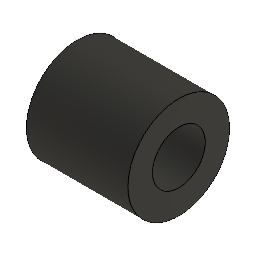
ServoBox (Autodesk Fusion 360 archive; units mm, degrees)
design "0.375 OD Spacer, 0.375 (Nylon)"
Autodesk Fusion 360 part; units mm, degrees
note: some values were not read from the file. Chosen so that the rebuilt part matches the saved one: a direction; which face or edge a step refers to. Set by a fixed rule: which sketch regions a step uses.
(part 1 of 2)
sketch "sketch 165" plane through (0, 0, 0) normal (1, 0, 0) x (0, 1, 0)
  circle A0 centre (0, 0) radius 4.7625
  circle A1 centre (0, 0) radius 2.4638
extrude "Extrude1" add sketch "sketch 165" along normal blind 9.525

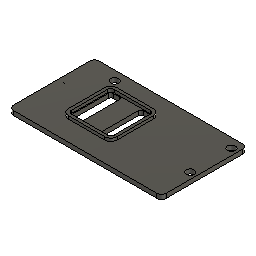
design "Encoder Mount"
Autodesk Fusion 360 part; units mm, degrees
sketch "Sketch1" plane through (0, 0, 0) normal (0, 0, 1) x (1, 0, 0)
  circle A0 centre (18.7728, 42.4051) radius 2.159
  line L0 (-60.9197, 30.0451) -> (-60.9197, 58.9153)
  line L1 (22.2603, 30.0451) -> (22.2603, 58.9153)
  circle A1 centre (-44.7272, 19.9053) radius 2.159
  circle A2 centre (18.7728, 19.9051) radius 2.159
  line L2 (-60.9197, 30.0451) -> (-60.9197, 17.3451)
  line L3 (22.2603, 30.0451) -> (22.2603, 17.3451)
  line L4 (19.7203, 14.8051) -> (3.2103, 14.8051)
  line L5 (-41.8697, 14.8051) -> (-58.3797, 14.8051)
  arc A3 (-60.9197, 17.3451) -> (-58.3797, 14.8051) centre (-58.3797, 17.3451) ccw
  arc A4 (19.7203, 14.8051) -> (22.2603, 17.3451) centre (19.7203, 17.3451) ccw
  line L6 (-41.8697, 14.8051) -> (3.2103, 14.8051)
  line L7 (-57.4272, 61.4553) -> (19.7203, 61.4553)
  line L8 (-57.4272, 61.4553) -> (-58.3797, 61.4553)
  arc A5 (-58.3797, 61.4553) -> (-60.9197, 58.9153) centre (-58.3797, 58.9153) ccw
  arc A6 (22.2603, 58.9153) -> (19.7203, 61.4553) centre (19.7203, 58.9153) ccw
  line L9 (-23.0468, 48.4378) -> (-19.6337, 48.4378)
  line L10 (-18.3637, 47.1678) -> (-18.3637, 27.4828)
  line L11 (-40.5887, 27.4828) -> (-40.5887, 47.1678)
  line L12 (-39.3187, 48.4378) -> (-35.9056, 48.4378)
  line L13 (-57.7726, 34.7366) -> (-57.0819, 34.7366)
  line L14 (-34.6356, 38.3051) -> (-34.6356, 47.1678)
  line L15 (-34.6356, 38.3051) -> (-34.6356, 27.4828)
  line L16 (-24.3168, 38.3051) -> (-24.3168, 47.1678)
  line L17 (-24.3168, 38.3051) -> (-24.3168, 27.4828)
  line L18 (-19.6337, 26.2128) -> (-23.0468, 26.2128)
  line L19 (-35.9056, 26.2128) -> (-39.3187, 26.2128)
  arc A7 (-39.3187, 48.4378) -> (-40.5887, 47.1678) centre (-39.3187, 47.1678) ccw
  arc A8 (-34.6356, 47.1678) -> (-35.9056, 48.4378) centre (-35.9056, 47.1678) ccw
  arc A9 (-23.0468, 48.4378) -> (-24.3168, 47.1678) centre (-23.0468, 47.1678) ccw
  arc A10 (-18.3637, 47.1678) -> (-19.6337, 48.4378) centre (-19.6337, 47.1678) ccw
  arc A11 (-19.6337, 26.2128) -> (-18.3637, 27.4828) centre (-19.6337, 27.4828) ccw
  arc A12 (-24.3168, 27.4828) -> (-23.0468, 26.2128) centre (-23.0468, 27.4828) ccw
  arc A13 (-35.9056, 26.2128) -> (-34.6356, 27.4828) centre (-35.9056, 27.4828) ccw
  arc A14 (-40.5887, 27.4828) -> (-39.3187, 26.2128) centre (-39.3187, 27.4828) ccw
  line L20 (-40.5887, 37.3253) -> (-60.9087, 37.3253)
  line L21 (-37.6121, 48.4378) -> (-37.6121, 61.4553)
  arc A15 (-57.0819, 34.7366) -> (-57.7726, 34.7366) centre (-57.4272, 32.6053) ccw
  point P0 (-54.3297, 57.5051)
  point P1 (-60.9197, 27.5051)
  point P2 (-60.9197, 71.9551)
  point P3 (22.2603, 27.5051)
  point P4 (22.2603, 71.9551)
  point P5 (-60.9197, 14.8051)
  point P6 (22.2603, 14.8051)
  point P7 (-18.3637, 48.4378)
  point P8 (-18.3637, 26.2128)
  point P9 (-40.5887, 26.2128)
  point P10 (-40.5887, 48.4378)
  dimension "d37" = 4.318
  dimension "d42" = 4.318
  dimension "d49" = 44.45
  dimension "d51" = 44.45
  dimension "d84" = 4.318
  dimension "d86" = 4.318
  dimension "d89" = 15.24
  dimension "d90" = 15.24
  dimension "d93" = 2.54
  dimension "d139" = 2.54
  dimension "d142" = 22.225
  dimension "d143" = 22.225
  dimension "d144" = 22.225
  dimension "d146" = 10.3188
  dimension "d149" = 1.27
  dimension "d155" = 20.32
  dimension "d156" = 13.0175
  constraint coincident P2 L0
  constraint coincident P4 L1
  constraint coincident P3 L1
  constraint coincident P1 L0
  constraint collinear L4 L5
  constraint coincident P5 L2
  constraint coincident P5 L5
  constraint tangent L2 A3
  constraint tangent L5 A3
  constraint coincident P6 L3
  constraint coincident P6 L4
  constraint tangent L3 A4
  constraint tangent L4 A4
  constraint equal A3 A4
  constraint perpendicular L0 L13
  constraint perpendicular L1 L7
  constraint perpendicular L0 L8
  constraint tangent L8 A5
  constraint tangent L0 A5
  constraint tangent L7 A6
  constraint tangent L1 A6
  constraint equal A5 A6
  constraint perpendicular L9 L10
  constraint perpendicular L10 L18
  constraint perpendicular L11 L18
  constraint perpendicular L7 L14
  constraint perpendicular L6 L15
  constraint perpendicular L7 L16
  constraint perpendicular L6 L17
  constraint collinear L18 L19
  constraint coincident P10 L11
  constraint coincident P10 L12
  constraint tangent L11 A7
  constraint tangent L12 A7
  constraint tangent L14 A8
  constraint tangent L12 A8
  constraint equal A7 A8
  constraint tangent L16 A9
  constraint tangent L9 A9
  constraint equal A7 A9
  constraint coincident P7 L9
  constraint coincident P7 L10
  constraint tangent L9 A10
  constraint tangent L10 A10
  constraint equal A7 A10
  constraint coincident P8 L10
  constraint coincident P8 L18
  constraint tangent L10 A11
  constraint tangent L18 A11
  constraint equal A7 A11
  constraint tangent L18 A12
  constraint tangent L17 A12
  constraint equal A7 A12
  constraint tangent L19 A13
  constraint tangent L15 A13
  constraint equal A7 A13
  constraint coincident P9 L19
  constraint coincident P9 L11
  constraint tangent L19 A14
  constraint tangent L11 A14
  constraint equal A7 A14
  constraint midpoint L11 L20.start
  constraint perpendicular L0 L20
  constraint midpoint L12 L21.start
  constraint perpendicular L7 L21
  constraint coincident L7 L21.end
  measures "d37" diameter of A0
  measures "d42" diameter of A15
  measures "d49" distance of P1 P2
  measures "d51" distance of P3 P4
  measures "d84" diameter of A1
  measures "d86" diameter of A2
  measures "d89" distance of L0.start P5
  measures "d90" distance of L1.start P6
  measures "d93" radius of A3
  measures "d139" radius of A5
  measures "d142" distance of P7 P8
  measures "d143" distance of P8 P9
  measures "d144" distance of P9 P10
  measures "d146" distance of L16.start L14.start
  measures "d149" radius of A7
  measures "d155" distance of L20.start L20.end
  measures "d156" distance of L21.start L21.end
extrude "Extrude11" add sketch "Sketch1" along normal blind 2.3813
sketch "Sketch10" plane through (0, 0, 2.3813) normal (0, 0, 1) x (-1, 0, 0)
  circle A0 centre (44.7272, -19.9053) radius 2.159
  circle A1 centre (-18.7728, -19.9051) radius 2.159
  circle A2 centre (-18.7728, -42.4051) radius 2.159
  line L0 (24.3168, -27.4828) -> (24.3168, -47.1678)
  line L1 (23.0468, -48.4378) -> (19.6337, -48.4378)
  line L2 (18.3637, -47.1678) -> (18.3637, -27.4828)
  line L3 (35.9056, -26.2128) -> (39.3187, -26.2128)
  line L4 (34.6356, -47.1678) -> (34.6356, -27.4828)
  line L5 (40.5887, -27.4828) -> (40.5887, -47.1678)
  line L6 (39.3187, -48.4378) -> (35.9056, -48.4378)
  line L7 (-22.2603, -17.3451) -> (-22.2603, -58.9153)
  arc A3 (-22.2603, -58.9153) -> (-19.7203, -61.4553) centre (-19.7203, -58.9153) ccw
  line L8 (-19.7203, -61.4553) -> (58.3797, -61.4553)
  arc A4 (58.3797, -61.4553) -> (60.9197, -58.9153) centre (58.3797, -58.9153) ccw
  line L9 (60.9197, -58.9153) -> (60.9197, -17.3451)
  arc A5 (60.9197, -17.3451) -> (58.3797, -14.8051) centre (58.3797, -17.3451) ccw
  line L10 (58.3797, -14.8051) -> (-19.7203, -14.8051)
  arc A6 (-19.7203, -14.8051) -> (-22.2603, -17.3451) centre (-19.7203, -17.3451) ccw
  arc A7 (39.3187, -48.4378) -> (40.5887, -47.1678) centre (39.3187, -47.1678) ccw
  arc A8 (34.6356, -47.1678) -> (35.9056, -48.4378) centre (35.9056, -47.1678) ccw
  arc A9 (35.9056, -26.2128) -> (34.6356, -27.4828) centre (35.9056, -27.4828) ccw
  arc A10 (40.5887, -27.4828) -> (39.3187, -26.2128) centre (39.3187, -27.4828) ccw
  arc A11 (23.0468, -48.4378) -> (24.3168, -47.1678) centre (23.0468, -47.1678) ccw
  arc A12 (18.3637, -47.1678) -> (19.6337, -48.4378) centre (19.6337, -47.1678) ccw
  arc A13 (19.6337, -26.2128) -> (18.3637, -27.4828) centre (19.6337, -27.4828) ccw
  line L11 (19.6337, -26.2128) -> (23.0468, -26.2128)
  arc A14 (24.3168, -27.4828) -> (23.0468, -26.2128) centre (23.0468, -27.4828) ccw
  line L12 (39.3264, -48.4391) -> (19.6414, -48.4391)
  line L13 (18.3714, -47.1691) -> (18.3714, -27.4841)
  line L14 (19.6414, -26.2141) -> (39.3264, -26.2141)
  line L15 (40.5964, -27.4841) -> (40.5964, -47.1691)
  arc A15 (39.3264, -48.4391) -> (40.5964, -47.1691) centre (39.3264, -47.1691) ccw
  arc A16 (18.3714, -47.1691) -> (19.6414, -48.4391) centre (19.6414, -47.1691) ccw
  arc A17 (19.6414, -26.2141) -> (18.3714, -27.4841) centre (19.6414, -27.4841) ccw
  arc A18 (40.5964, -27.4841) -> (39.3264, -26.2141) centre (39.3264, -27.4841) ccw
  line L16 (19.6414, -25.6849) -> (39.3264, -25.6849)
  arc A19 (41.1255, -27.4841) -> (39.3264, -25.6849) centre (39.3264, -27.4841) ccw
  line L17 (41.1255, -27.4841) -> (41.1255, -47.1691)
  arc A20 (39.3264, -48.9683) -> (41.1255, -47.1691) centre (39.3264, -47.1691) ccw
  line L18 (39.3264, -48.9683) -> (19.6414, -48.9683)
  arc A21 (17.8422, -47.1691) -> (19.6414, -48.9683) centre (19.6414, -47.1691) ccw
  line L19 (17.8422, -47.1691) -> (17.8422, -27.4841)
  arc A22 (19.6414, -25.6849) -> (17.8422, -27.4841) centre (19.6414, -27.4841) ccw
  arc A23 (16.2547, -47.1691) -> (19.6414, -50.5558) centre (19.6414, -47.1691) ccw
  line L20 (39.3264, -50.5558) -> (19.6414, -50.5558)
  arc A24 (39.3264, -50.5558) -> (42.713, -47.1691) centre (39.3264, -47.1691) ccw
  line L21 (42.713, -27.4841) -> (42.713, -47.1691)
  arc A25 (42.713, -27.4841) -> (39.3264, -24.0974) centre (39.3264, -27.4841) ccw
  line L22 (19.6414, -24.0974) -> (39.3264, -24.0974)
  arc A26 (19.6414, -24.0974) -> (16.2547, -27.4841) centre (19.6414, -27.4841) ccw
  line L23 (16.2547, -47.1691) -> (16.2547, -27.4841)
  arc A27 (57.0819, -34.7366) -> (57.7726, -34.7366) centre (57.4272, -32.6053) ccw
  line L24 (57.0819, -34.7366) -> (57.7726, -34.7366)
  dimension "d150" = -0.5292
  dimension "d151" = 1.27
  dimension "d154" = -1.5875
  constraint perpendicular L2 L12
  constraint perpendicular L11 L13
  constraint perpendicular L5 L14
  constraint perpendicular L12 L15
  constraint tangent L12 A15
  constraint tangent L15 A15
  constraint tangent L12 A16
  constraint tangent L13 A16
  constraint equal A15 A16
  constraint tangent L13 A17
  constraint tangent L14 A17
  constraint equal A15 A17
  constraint tangent L14 A18
  constraint tangent L15 A18
  constraint equal A15 A18
  measures "d151" radius of A15
extrude "Extrude12" add sketch "Sketch10" against normal blind 3.9688 contours A23 L20 A24 L21 A25 L22 A26 L23
move_body "Move1" bodies 1 to x (1, 0, 0) y (0, -1, 0) z (0, 0, -1) at (0, 51.5532, 4.7625)
equation "d142 = ( 7 / 8 ) * 1 in"
equation "d143 = ( 7 / 8 ) * 1 in"
equation "d144 = ( 7 / 8 ) * 1 in"
equation "d146 = ( 13 / 32 ) * 1 in"
equation "d147 = ( 3 / 32 ) * 1 in"
equation "d150 = ( -1 / 48 ) * 1 in"
equation "d152 = ( -5 / 32 ) * 1 in"
equation "d154 = ( -1 / 16 ) * 1 in"
equation "d120 = ( 3 / 16 ) * 1 in"
equation "d122 = 2.04724 in + 0.375 in"
equation "d123 = ( 3 / 16 ) * 1 in"
equation "d130 = -( 3 / 16 ) * 1 in"
equation "d134 = cm"
named bodies: "EncoderMount"

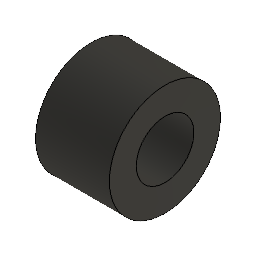
design "0.375 OD Spacer, 0.250 (Nylon)"
Autodesk Fusion 360 part; units mm, degrees
sketch "sketch 165" plane through (0, 0, 0) normal (1, 0, 0) x (0, 1, 0)
  circle A0 centre (0, 0) radius 4.7625
  circle A1 centre (0, 0) radius 2.4638
extrude "Extrude1" add sketch "sketch 165" along normal blind 6.35

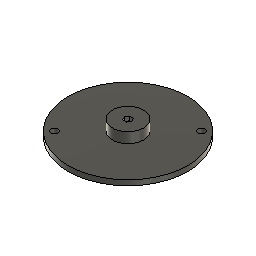
design "Winch2"
Autodesk Fusion 360 part; units mm, degrees
sketch "Sketch1" plane through (0, 0, 0) normal (0, 0, 1) x (1, 0, 0)
  circle A0 centre (0, 0) radius 18.2563
  line L0 (0, 0) -> (18.2563, 0) construction
  circle A1 centre (22.4506, 22.4506) radius 2.159
  circle A2 centre (-22.4506, -22.4506) radius 2.159
  circle A3 centre (0, 0) radius 9.525
  circle A4 centre (0, 0) radius 36.5125
  circle A5 centre (0, 0) radius 31.75
  line L1 (0, 0) -> (22.4506, 22.4506)
  line L2 (0, 0) -> (21.082, 0) construction
  line L3 (0, 0) -> (-22.4506, -22.4506)
  line L4 (0, 0) -> (21.082, 0) construction
  dimension "d1" = 36.5125
  dimension "d16" = 4.318
  dimension "d18" = 4.318
  dimension "d24" = 19.05
  dimension "d33" = 73.025
  dimension "d34" = 63.5
  dimension "d35" = 45
  dimension "d36" = 135
  constraint coincident A0.centre L0.start
  constraint horizontal L0
  constraint concentric A0 A4
  constraint concentric A3 A5
  constraint horizontal L2
  constraint coincident A5 A1.centre
  constraint coincident A1.centre L1.end
  constraint horizontal L4
  constraint coincident A5 A2.centre
  constraint coincident A2.centre L3.end
  measures "d1" diameter of A0
  measures "d16" diameter of A1
  measures "d18" diameter of A2
  measures "d24" diameter of A3
  measures "d33" diameter of A4
  measures "d34" diameter of A5
  measures "d35" angle of L1 L2
  measures "d36" angle of L3 L4
extrude "Extrude2" add sketch "Sketch1" along normal blind 3.175 contours A0 A3 L1 L3 | A0 A3 L1 L3 | A3 L1 L3 | A3 L1 L3
sketch "Sketch2" plane through (0, 0, 3.175) normal (0, 0, 1) x (-1, 0, 0)
  circle A0 centre (0, 0) radius 18.2563
  circle A1 centre (0, 0) radius 9.525
  dimension "d27" = 19.05
  constraint coincident A0.centre A1.centre
  measures "d27" diameter of A1
extrude "Extrude3" add sketch "Sketch2" along normal blind 6.35 contours A1
sketch "Sketch3" plane through (0, 0, 9.525) normal (0, 0, 1) x (-1, 0, 0)
  circle A0 centre (0, 0) radius 9.525
  line L0 (-1.2943, -1.9151) -> (1.0113, -2.0784)
  line L1 (1.0113, -2.0784) -> (2.3056, -0.1633)
  line L2 (2.3056, -0.1633) -> (1.2943, 1.9151)
  line L3 (1.2943, 1.9151) -> (-1.0113, 2.0784)
  line L4 (-1.0113, 2.0784) -> (-2.3056, 0.1633)
  line L5 (-2.3056, 0.1633) -> (-1.2943, -1.9151)
  dimension "d42" = 2.3114
  constraint coincident A0.centre origin
  measures "d42" distance of L0.start A0.centre
extrude "Extrude7" add sketch "Sketch1" along normal blind 3.175 contours A0 A1 A2 A5 L1 L3 | A0 A1 A2 A5 L1 L3 | A4
extrude "Extrude8" cut sketch "Sketch3" against normal blind 2.3813 contours L0 L1 L2 L3 L4 L5
extrude "Extrude6" add sketch "Sketch1" along normal blind 3.175 contours A0 A1 A2 A5 L1 L3 | A0 A1 A2 A5 L1 L3 | A4
extrude "Extrude4" cut sketch "Sketch3" against normal blind 2.5 contours L0 L1 L2 L3 L4 L5
extrude "Extrude5" add sketch "Sketch1" along normal blind 3.175 contours A0 A1 A2 A5 L1 L3 | A0 A1 A2 A5 L1 L3 | A4
equation "d1 = ( 23 / 16 ) * 1 in"
equation "d45 = ( -3 / 32 ) * 1 in"
named bodies: "Winch2"

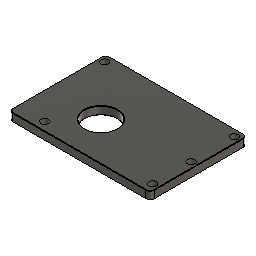
design "ServoPlate"
Autodesk Fusion 360 part; units mm, degrees
sketch "Sketch1" plane through (0, 0, 0) normal (0, 0, 1) x (1, 0, 0)
  circle A0 centre (18.7728, 42.4051) radius 2.159
  line L0 (-60.9197, 30.0451) -> (-60.9197, 69.4151)
  line L1 (22.2603, 30.0451) -> (22.2603, 69.4151)
  line L2 (19.7203, 71.9551) -> (-58.3797, 71.9551)
  arc A1 (-58.3797, 71.9551) -> (-60.9197, 69.4151) centre (-58.3797, 69.4151) ccw
  arc A2 (22.2603, 69.4151) -> (19.7203, 71.9551) centre (19.7203, 69.4151) ccw
  line L3 (-60.9197, 71.9551) -> (22.2603, 71.9551)
  circle A3 centre (-57.4272, 67.8053) radius 2.159
  circle A4 centre (18.7728, 67.8053) radius 2.159
  circle A5 centre (-44.7272, 19.9053) radius 2.159
  circle A6 centre (18.7728, 19.9051) radius 2.159
  line L4 (-60.9197, 30.0451) -> (-60.9197, 17.3451)
  line L5 (22.2603, 30.0451) -> (22.2603, 17.3451)
  line L6 (19.7203, 14.8051) -> (3.2103, 14.8051)
  line L7 (-41.8697, 14.8051) -> (-58.3797, 14.8051)
  arc A7 (-60.9197, 17.3451) -> (-58.3797, 14.8051) centre (-58.3797, 17.3451) ccw
  arc A8 (19.7203, 14.8051) -> (22.2603, 17.3451) centre (19.7203, 17.3451) ccw
  line L8 (-41.8697, 14.8051) -> (3.2103, 14.8051)
  line L9 (-60.9197, 34.7366) -> (-29.1697, 34.7366)
  line L10 (-28.759, 14.8051) -> (-28.759, 38.3051)
  circle A9 centre (-30.3427, 38.3051) radius 9.5885
  arc A10 (-57.0819, 34.7366) -> (-57.7726, 34.7366) centre (-57.4272, 32.6053) ccw
  point P0 (-54.3297, 57.5051)
  point P1 (-60.9197, 27.5051)
  point P2 (-60.9197, 71.9551)
  point P3 (22.2603, 27.5051)
  point P4 (22.2603, 71.9551)
  point P5 (-60.9197, 14.8051)
  point P6 (22.2603, 14.8051)
  dimension "d37" = 4.318
  dimension "d42" = 4.318
  dimension "d49" = 44.45
  dimension "d51" = 44.45
  dimension "d52" = 2.54
  dimension "d54" = 4.318
  dimension "d66" = 4.318
  dimension "d84" = 4.318
  dimension "d86" = 4.318
  dimension "d89" = 15.24
  dimension "d90" = 15.24
  dimension "d93" = 2.54
  dimension "d106" = 31.75
  dimension "d107" = 23.5
  dimension "d108" = 19.177
  constraint coincident P2 L0
  constraint coincident P2 L2
  constraint tangent L0 A1
  constraint tangent L2 A1
  constraint coincident P4 L1
  constraint coincident P4 L2
  constraint tangent L1 A2
  constraint tangent L2 A2
  constraint equal A1 A2
  constraint coincident P3 L1
  constraint coincident P1 L0
  constraint coincident P2 L3.start
  constraint coincident P4 L3.end
  constraint collinear L6 L7
  constraint coincident P5 L4
  constraint coincident P5 L7
  constraint tangent L4 A7
  constraint tangent L7 A7
  constraint coincident P6 L5
  constraint coincident P6 L6
  constraint tangent L5 A8
  constraint tangent L6 A8
  constraint equal A7 A8
  constraint coincident L0 L9.start
  constraint perpendicular L0 L9
  constraint coincident L8 L10.start
  constraint perpendicular L8 L10
  constraint coincident L9 A10.end
  constraint coincident L9 A10.start
  measures "d37" diameter of A0
  measures "d42" diameter of A10
  measures "d49" distance of P1 P2
  measures "d51" distance of P3 P4
  measures "d52" radius of A1
  measures "d54" diameter of A3
  measures "d66" diameter of A4
  measures "d84" diameter of A5
  measures "d86" diameter of A6
  measures "d89" distance of L0.start P5
  measures "d90" distance of L1.start P6
  measures "d93" radius of A7
  measures "d106" distance of L9.start L9.end
  measures "d107" distance of L10.start L10.end
  measures "d108" diameter of A9
extrude "Extrude4" add sketch "Sketch1" along normal blind 4.7625
fillet "Fillet5" radius 0.254 28 edges at (-60.9197, 32.3908, 0) (-60.9197, 32.3908, 4.7625) (-60.9197, 23.6951, 0) (-60.9197, 23.6951, 4.7625) (-60.1758, 15.549, 0) (-60.1758, 15.549, 4.7625) (-50.1247, 14.8051, 0) (-50.1247, 14.8051, 4.7625) (-35.3144, 14.8051, 0) (-35.3144, 14.8051, 4.7625) (-12.7744, 14.8051, 0) (-12.7744, 14.8051, 4.7625) (11.4653, 14.8051, 0) (11.4653, 14.8051, 4.7625) (21.5163, 15.549, 0) (21.5163, 15.549, 4.7625) (22.2603, 23.6951, 0) (22.2603, 23.6951, 4.7625) (22.2603, 49.7301, 0) (22.2603, 49.7301, 4.7625) (21.5163, 71.2111, 0) (21.5163, 71.2111, 4.7625) (-19.3297, 71.9551, 0) (-19.3297, 71.9551, 4.7625) (-60.1758, 71.2111, 0) (-60.1758, 71.2111, 4.7625) (-60.9197, 52.0758, 0) (-60.9197, 52.0758, 4.7625)
sketch "Sketch4" plane through (0, 0, 4.7625) normal (0, 0, 1) x (-1, 0, 0)
  circle A0 centre (44.7272, -19.9053) radius 2.159
  circle A1 centre (-18.7728, -42.4051) radius 2.159
  circle A2 centre (-18.7728, -67.8053) radius 2.159
  circle A3 centre (57.4272, -67.8053) radius 2.159
  circle A4 centre (-18.7728, -19.9051) radius 2.159
  line L0 (58.3797, -15.0591) -> (-19.7203, -15.0591)
  arc A5 (-19.7203, -15.0591) -> (-22.0063, -17.3451) centre (-19.7203, -17.3451) ccw
  line L1 (-22.0063, -17.3451) -> (-22.0063, -69.4151)
  arc A6 (-22.0063, -69.4151) -> (-19.7203, -71.7011) centre (-19.7203, -69.4151) ccw
  line L2 (-19.7203, -71.7011) -> (58.3797, -71.7011)
  arc A7 (58.3797, -71.7011) -> (60.6657, -69.4151) centre (58.3797, -69.4151) ccw
  line L3 (60.6657, -69.4151) -> (60.6657, -17.3451)
  arc A8 (60.6657, -17.3451) -> (58.3797, -15.0591) centre (58.3797, -17.3451) ccw
  line L4 (29.4237, -15.0591) -> (29.4237, -37.5591)
  circle A9 centre (29.4237, -37.5591) radius 9.5885
  line L5 (60.6657, -37.5591) -> (29.4237, -37.5591)
  dimension "d110" = 22.5
  dimension "d111" = 19.177
  dimension "d139" = 31.242
  constraint coincident L0 L4.start
  constraint perpendicular L0 L4
  constraint coincident L4.end A9.centre
  constraint coincident L3 L5.start
  constraint perpendicular L4 L5
  measures "d110" distance of L4.start L4.end
  measures "d111" diameter of A9
  measures "d139" distance of L5.start L4.end
extrude "Extrude6" cut sketch "Sketch4" against normal up to surface (4.7625 mm away) contours L4 A9 L5 | L4 A9 L5
fillet "Fillet7" radius 0.254 2 edges at (-20.4841, 41.0264, 0) (-20.4841, 34.0917, 4.7625)
sketch "Sketch5" plane through (0, 0, 4.7625) normal (0, 0, 1) x (-1, 0, 0)
  line L0 (58.3797, -15.0591) -> (-19.7203, -15.0591)
  arc A0 (-19.7203, -15.0591) -> (-22.0063, -17.3451) centre (-19.7203, -17.3451) ccw
  line L1 (-22.0063, -17.3451) -> (-22.0063, -69.4151)
  arc A1 (-22.0063, -69.4151) -> (-19.7203, -71.7011) centre (-19.7203, -69.4151) ccw
  line L2 (-19.7203, -71.7011) -> (58.3797, -71.7011)
  arc A2 (58.3797, -71.7011) -> (60.6657, -69.4151) centre (58.3797, -69.4151) ccw
  line L3 (60.6657, -69.4151) -> (60.6657, -17.3451)
  arc A3 (60.6657, -17.3451) -> (58.3797, -15.0591) centre (58.3797, -17.3451) ccw
  circle A4 centre (-18.7728, -19.9051) radius 2.159
  circle A5 centre (57.4272, -67.8053) radius 2.159
  circle A6 centre (-18.7728, -67.8053) radius 2.159
  circle A7 centre (-18.7728, -42.4051) radius 2.159
  circle A8 centre (44.7272, -19.9053) radius 2.159
  circle A9 centre (29.4237, -37.5591) radius 9.8425
  line L4 (-18.7728, -42.4051) -> (-18.7728, -48.7551)
  line L5 (-22.0063, -48.7551) -> (-16.9198, -48.7551)
  line L6 (-18.7728, -32.6051) -> (-18.7728, -26.2551)
  line L7 (-14.3798, -46.2151) -> (-14.3798, -28.7904)
  line L8 (-16.9198, -26.2504) -> (-22.0063, -26.2504)
  arc A10 (-16.9198, -48.7551) -> (-14.3798, -46.2151) centre (-16.9198, -46.2151) ccw
  line L9 (-22.0063, -48.7551) -> (-22.2606, -48.7551)
  line L10 (-22.0063, -26.2504) -> (-22.2606, -26.2504)
  arc A11 (-14.3798, -28.7904) -> (-16.9198, -26.2504) centre (-16.9198, -28.7904) ccw
  line L11 (-22.2606, -48.7551) -> (-22.2606, -26.2504)
  dimension "d116" = 6.35
  dimension "d117" = 6.35
  dimension "d118" = 2.54
  dimension "d119" = 2.54
  constraint coincident A7.centre L4.start
  constraint parallel L1 L4
  constraint coincident L1 L5.start
  constraint perpendicular L4 L5
  constraint parallel L1 L6
  constraint perpendicular L5 L7
  constraint coincident L1 L8.end
  constraint perpendicular L1 L8
  constraint tangent L5 A10
  constraint tangent L7 A10
  constraint perpendicular L1 L9
  constraint perpendicular L1 L10
  constraint tangent L7 A11
  constraint tangent L8 A11
  constraint perpendicular L10 L11
  measures "d116" distance of A7.centre L4.end
  measures "d117" distance of L6.start L6.end
  measures "d118" radius of A10
  measures "d119" radius of A11
sketch "Sketch6" plane through (22.2606, 0, 0) normal (1, 0, 0) x (0, 1, 0)
  line L0 (26.2504, 4.7625) -> (48.7551, 4.7625)
  line L1 (48.7551, 4.7625) -> (48.7551, 9.525)
  line L2 (48.7551, 9.525) -> (26.2504, 9.525)
  line L3 (26.2504, 9.525) -> (26.2504, 4.7625)
sketch "Sketch7" plane through (22.2606, 0, 0) normal (1, 0, 0) x (0, 1, 0)
  line L0 (26.2504, 9.5249) -> (48.7567, 9.5249)
  line L1 (48.7567, 9.5249) -> (48.7567, -52)
  line L2 (48.7567, -52) -> (26.2504, -52)
  line L3 (26.2504, -52) -> (26.2504, 9.5249)
  dimension "d122" = 61.5249
  constraint horizontal L0
  constraint vertical L1
  constraint horizontal L2
  constraint vertical L3
  measures "d122" distance of L0.start L2.end
sketch "Sketch8" plane through (0, 0, -52) normal (0, 0, -1) x (1, 0, 0)
  line L0 (22.2606, -26.2504) -> (22.2606, -48.7567)
  line L1 (22.2606, -48.7567) -> (27.0231, -48.7567)
  line L2 (27.0231, -48.7567) -> (27.0231, -26.2504)
  line L3 (27.0231, -26.2504) -> (22.2606, -26.2504)
  line L4 (22.2606, -26.2504) -> (17.1806, -26.2504)
  line L5 (22.2606, -48.7567) -> (17.1806, -48.7567)
  line L6 (14.6406, -46.2167) -> (14.6406, -28.7904)
  arc A0 (17.1806, -26.2504) -> (14.6406, -28.7904) centre (17.1806, -28.7904) ccw
  arc A1 (14.6406, -46.2167) -> (17.1806, -48.7567) centre (17.1806, -46.2167) ccw
  line L7 (18.7728, -48.7551) -> (18.7728, -26.2504)
  circle A2 centre (18.7728, -42.4051) radius 2.159
  circle A3 centre (18.7728, -32.6051) radius 2.159
  point P0 (14.6406, -26.2504)
  point P1 (14.6406, -48.7567)
  dimension "d125" = 7.62
  dimension "d126" = 7.62
  dimension "d127" = 2.54
  dimension "d128" = 4.318
  dimension "d129" = 4.318
  constraint coincident L0.start L3.end
  constraint perpendicular L0 L4
  constraint coincident L0.end L1.start
  constraint perpendicular L0 L5
  constraint coincident P0 L4
  constraint coincident P0 L6
  constraint tangent L4 A0
  constraint tangent L6 A0
  constraint coincident P1 L5
  constraint coincident P1 L6
  constraint tangent L5 A1
  constraint tangent L6 A1
  constraint equal A0 A1
  constraint coincident L4 L7.end
  constraint perpendicular L4 L7
  constraint coincident L7 A2.centre
  constraint coincident L7 A3.centre
  measures "d125" distance of L0.start P0
  measures "d126" distance of L0.end P1
  measures "d127" radius of A0
  measures "d128" diameter of A2
  measures "d129" diameter of A3
sketch "Sketch9" plane through (27.0231, 0, 0) normal (1, 0, 0) x (0, 1, 0)
  line L0 (26.2504, -52) -> (48.7567, -52)
  line L1 (48.7567, -52) -> (48.7567, 9.5249)
  line L2 (48.7567, 9.5249) -> (26.2504, 9.5249)
  line L3 (26.2504, 9.5249) -> (26.2504, -52)
  line L4 (26.2504, -21.2375) -> (48.7567, -21.2375)
  line L5 (37.5036, -52) -> (37.5036, 9.5249)
  line L6 (37.5036, 9.5249) -> (37.5036, -15.8751)
  line L7 (37.5036, -15.8751) -> (27.5036, -15.8751)
  line L8 (37.5036, -15.8751) -> (47.5036, -15.8751)
  circle A0 centre (42.5036, -15.8751) radius 2.5
  circle A1 centre (32.5036, -15.8751) radius 2.5
  dimension "d132" = 25.4
  dimension "d133" = 10
  dimension "d134" = 10
  dimension "d135" = 5
  dimension "d136" = 5
  constraint midpoint L3 L4.start
  constraint midpoint L1 L4.end
  constraint midpoint L0 L5.start
  constraint midpoint L2 L5.end
  constraint coincident L5 L6.end
  constraint perpendicular L5 L7
  constraint perpendicular L1 L8
  constraint midpoint L8 A0.centre
  constraint midpoint L7 A1.centre
  measures "d132" distance of L5.end L6.end
  measures "d133" distance of L6.end L7.end
  measures "d134" distance of L6.end L8.end
  measures "d135" diameter of A0
  measures "d136" diameter of A1
equation "d94 = ( 3 / 16 ) * 1 in"
equation "d122 = 2.04724 in + 0.375 in"
equation "d134 = cm"
named bodies: "ServoPlate"

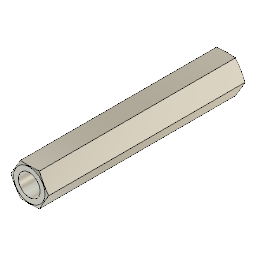
design "1.500 Standoff (8-32, Aluminum)"
Autodesk Fusion 360 part; units mm, degrees
sketch "sketch 165" plane through (0, 0, 0) normal (0, 1, 0) x (-1, 0, 0)
  line L0 (3.6662, 0) -> (1.8331, 3.175)
  line L1 (0, 3.175) -> (-1.8331, 3.175)
  line L2 (-1.8331, 3.175) -> (-3.6662, 0)
  line L3 (-3.6662, 0) -> (-1.8331, -3.175)
  line L4 (-1.8331, -3.175) -> (0, -3.175)
  line L5 (0, -3.175) -> (1.8331, -3.175)
  line L6 (1.8331, -3.175) -> (3.6662, 0)
  line L7 (3.6662, 0) -> (1.8331, 3.175)
  line L8 (1.8331, 3.175) -> (0, 3.175)
  circle A0 centre (0, 0) radius 2.0955
extrude "Extrude1" add sketch "sketch 165" along normal blind 38.1 contours L0 L1 L2 L3 L4 L5 L6 L7 L8 | A0
extrude "Extrude2" cut sketch "sketch 165" along normal blind 12.7 contours A0
extrude "Extrude3" cut sketch "sketch 165" against normal blind 12.7 from surface at 38.1 contours A0
ref_plane "WorkPlane1" through (19.05, 0, 0) normal (1, 0, 0) x (0, 1, 0)
sketch "Sketch1" plane through (0, 0, 0) normal (1, 0, 0) x (0, 1, 0)
  arc A0 (0, -3.0312) -> (0.127, -3.6662) centre (1.651, -3.0312) ccw
  line L0 (0.127, -3.6662) -> (0, -3.6662)
  line L1 (0, -3.6662) -> (0, -3.0312)
  line L2 (0, 0) -> (0, -3.0312) construction
  line L3 (19.05, -3.175) -> (19.05, 3.175) construction
  line L4 (38.1, -3.6662) -> (38.1, -3.0312)
  line L5 (37.973, -3.6662) -> (38.1, -3.6662)
  arc A1 (37.973, -3.6662) -> (38.1, -3.0312) centre (36.449, -3.0312) ccw
  line L6 (0, 0) -> (19.05, 0) construction
  dimension "d8" = 1.651
  dimension "d9" = 0.635
  dimension "d11" = 3.0312
  dimension "d13" = 19.05
  dimension "d14" = 6.35
  constraint horizontal L0
  constraint tangent A0 L1
  constraint coincident L2.start L6.start
  constraint tangent A0 L2
  constraint vertical L2
  constraint vertical L3
  constraint symmetric A0.end L3 L5.start
  constraint symmetric A0.start L3 L4.end
  constraint symmetric A0 L3 A1
  constraint symmetric L0.end L3 L4.start
  constraint midpoint L3 L6.end
  constraint horizontal L6
  measures "d8" radius of A0
  measures "d9" vertical distance of A0.end A0.start
  measures "d11" distance of L2.start A0.start
  measures "d13" distance of L2.start L3
  measures "d14" distance of L3.start L3.end
revolve "Revolve1" cut sketch "Sketch1" angle 360 about axis through (0, 0, 0) along (0, 1, 0)
equation "length_distance = 1.500 in"
equation "d3 = min(length_distance / 2; 0.5 in)"
equation "d6 = -min(length_distance / 2; 0.5 in)"
equation "d12 = length_distance / 2"
equation "d13 = length_distance / 2"

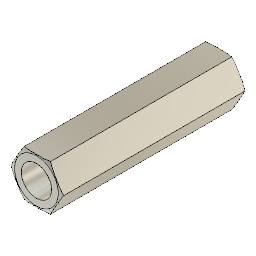
design "1.000 Standoff (8-32, Aluminum)"
Autodesk Fusion 360 part; units mm, degrees
sketch "sketch 165" plane through (0, 0, 0) normal (0, 1, 0) x (-1, 0, 0)
  line L0 (3.6662, 0) -> (1.8331, 3.175)
  line L1 (0, 3.175) -> (-1.8331, 3.175)
  line L2 (-1.8331, 3.175) -> (-3.6662, 0)
  line L3 (-3.6662, 0) -> (-1.8331, -3.175)
  line L4 (-1.8331, -3.175) -> (0, -3.175)
  line L5 (0, -3.175) -> (1.8331, -3.175)
  line L6 (1.8331, -3.175) -> (3.6662, 0)
  line L7 (3.6662, 0) -> (1.8331, 3.175)
  line L8 (1.8331, 3.175) -> (0, 3.175)
  circle A0 centre (0, 0) radius 2.0955
extrude "Extrude1" add sketch "sketch 165" along normal blind 25.4 contours L0 L1 L2 L3 L4 L5 L6 L7 L8 | A0
extrude "Extrude2" cut sketch "sketch 165" along normal blind 12.7 contours A0
extrude "Extrude3" cut sketch "sketch 165" against normal blind 12.7 from surface at 25.4 contours A0
ref_plane "WorkPlane1" through (12.7, 0, 0) normal (1, 0, 0) x (0, 1, 0)
sketch "Sketch1" plane through (0, 0, 0) normal (1, 0, 0) x (0, 1, 0)
  arc A0 (0, -3.0312) -> (0.127, -3.6662) centre (1.651, -3.0312) ccw
  line L0 (0.127, -3.6662) -> (0, -3.6662)
  line L1 (0, -3.6662) -> (0, -3.0312)
  line L2 (0, 0) -> (0, -3.0312) construction
  line L3 (12.7, -3.175) -> (12.7, 3.175) construction
  line L4 (25.4, -3.6662) -> (25.4, -3.0312)
  line L5 (25.273, -3.6662) -> (25.4, -3.6662)
  arc A1 (25.273, -3.6662) -> (25.4, -3.0312) centre (23.749, -3.0312) ccw
  line L6 (0, 0) -> (12.7, 0) construction
  dimension "d8" = 1.651
  dimension "d9" = 0.635
  dimension "d11" = 3.0312
  dimension "d13" = 12.7
  dimension "d14" = 6.35
  constraint horizontal L0
  constraint tangent A0 L1
  constraint coincident L2.start L6.start
  constraint tangent A0 L2
  constraint vertical L2
  constraint vertical L3
  constraint symmetric A0.end L3 L5.start
  constraint symmetric A0.start L3 L4.end
  constraint symmetric A0 L3 A1
  constraint symmetric L0.end L3 L4.start
  constraint midpoint L3 L6.end
  constraint horizontal L6
  measures "d8" radius of A0
  measures "d9" vertical distance of A0.end A0.start
  measures "d11" distance of L2.start A0.start
  measures "d13" distance of L2.start L3
  measures "d14" distance of L3.start L3.end
revolve "Revolve1" cut sketch "Sketch1" angle 360 about axis through (0, 0, 0) along (0, 1, 0)
equation "length_distance = 1.00 in"
equation "d3 = min(length_distance / 2; 0.5 in)"
equation "d6 = -min(length_distance / 2; 0.5 in)"
equation "d12 = length_distance / 2"
equation "d13 = length_distance / 2"

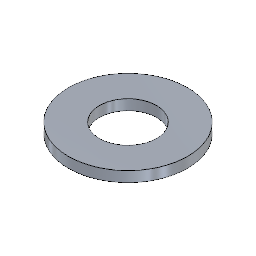
design "Small Washer, 0.03125 (Steel)"
Autodesk Fusion 360 part; units mm, degrees
sketch "Sketch1" plane through (0, 0, 0) normal (0, 0, 1) x (1, 0, 0)
  circle A0 centre (0, 0) radius 2.1463
  circle A1 centre (0, 0) radius 4.4958
  dimension "d1" = 4.2926
  dimension "d2" = 8.9916
  constraint coincident A0.centre A1.centre
  constraint concentric A0 A1
  measures "d1" diameter of A0
  measures "d2" diameter of A1
extrude "Extrude1" add sketch "Sketch1" along normal blind 0.7937
equation "d3 = ( 1 / 32 ) * 1 in"

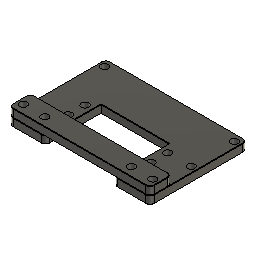
design "ServoMount"
Autodesk Fusion 360 part; units mm, degrees
sketch "Sketch1" plane through (0, 0, 0) normal (0, 0, 1) x (1, 0, 0)
  line L0 (-39.3297, 47.5051) -> (-1.8697, 47.5051)
  line L1 (0.6703, 44.9651) -> (0.6703, 30.0451)
  line L2 (-39.3297, 44.9651) -> (-39.3297, 30.0451)
  line L3 (-36.7897, 47.5051) -> (0.6703, 47.5051)
  circle A0 centre (-43.6297, 42.4053) radius 2.159
  circle A1 centre (4.9703, 42.4051) radius 2.159
  circle A2 centre (-43.6297, 32.6053) radius 2.159
  circle A3 centre (4.9703, 32.6051) radius 2.159
  line L4 (-39.3297, 47.5051) -> (-39.3297, 44.9651)
  line L5 (0.6703, 47.5051) -> (0.6703, 44.9651)
  line L6 (-60.9197, 30.0451) -> (-60.9197, 69.4151)
  line L7 (22.2603, 30.0451) -> (22.2603, 69.4151)
  line L8 (19.7203, 71.9551) -> (-58.3797, 71.9551)
  arc A4 (-58.3797, 71.9551) -> (-60.9197, 69.4151) centre (-58.3797, 69.4151) ccw
  arc A5 (22.2603, 69.4151) -> (19.7203, 71.9551) centre (19.7203, 69.4151) ccw
  line L9 (-60.9197, 71.9551) -> (22.2603, 71.9551)
  circle A6 centre (-57.4272, 67.8053) radius 2.159
  circle A7 centre (18.7728, 67.8053) radius 2.159
  circle A8 centre (-57.4272, 19.9053) radius 2.159
  circle A9 centre (-44.7272, 19.9053) radius 2.159
  circle A10 centre (18.7728, 19.9051) radius 2.159
  circle A11 centre (6.0728, 19.9051) radius 2.159
  line L10 (-60.9197, 30.0451) -> (-60.9197, 17.3451)
  line L11 (22.2603, 30.0451) -> (22.2603, 17.3451)
  line L12 (-39.3297, 30.0451) -> (-39.3297, 17.3451)
  line L13 (0.6703, 30.0451) -> (0.6703, 17.3451)
  line L14 (19.7203, 14.8051) -> (3.2103, 14.8051)
  line L15 (-41.8697, 14.8051) -> (-58.3797, 14.8051)
  arc A12 (-60.9197, 17.3451) -> (-58.3797, 14.8051) centre (-58.3797, 17.3451) ccw
  arc A13 (-41.8697, 14.8051) -> (-39.3297, 17.3451) centre (-41.8697, 17.3451) ccw
  arc A14 (0.6703, 17.3451) -> (3.2103, 14.8051) centre (3.2103, 17.3451) ccw
  arc A15 (19.7203, 14.8051) -> (22.2603, 17.3451) centre (19.7203, 17.3451) ccw
  circle A16 centre (-30.1476, 67.8053) radius 2.159
  circle A17 centre (-2.868, 67.8053) radius 2.159
  line L16 (-57.4272, 67.8053) -> (-19.3272, 67.8053)
  circle A18 centre (4.9703, 42.4051) radius 2.159
  line L17 (18.7728, 67.8053) -> (18.7728, 19.9051)
  circle A19 centre (4.9703, 42.4051) radius 2.159
  circle A20 centre (4.9703, 42.4051) radius 2.159
  line L18 (4.9703, 42.4051) -> (4.9703, 71.9551)
  line L19 (4.9703, 42.4051) -> (18.7728, 42.4051)
  circle A21 centre (18.7728, 42.4051) radius 2.159
  line L20 (18.7728, 42.4051) -> (-57.4272, 42.4051)
  point P0 (-54.3297, 57.5051)
  point P1 (-60.9197, 27.5051)
  point P2 (-60.9197, 71.9551)
  point P3 (22.2603, 27.5051)
  point P4 (22.2603, 71.9551)
  point P5 (-60.9197, 14.8051)
  point P6 (22.2603, 14.8051)
  dimension "d11" = 4.318
  dimension "d14" = 4.318
  dimension "d15" = 9.8
  dimension "d16" = 4.318
  dimension "d17" = 9.8
  dimension "d18" = 4.318
  dimension "d49" = 44.45
  dimension "d51" = 44.45
  dimension "d52" = 2.54
  dimension "d54" = 4.318
  dimension "d66" = 4.318
  dimension "d82" = 4.318
  dimension "d84" = 4.318
  dimension "d86" = 4.318
  dimension "d88" = 4.318
  dimension "d89" = 15.24
  dimension "d90" = 15.24
  dimension "d93" = 2.54
  dimension "d108" = 54.5592
  dimension "d109" = 0
  dimension "d110" = 38.1
  dimension "d112" = 4.318
  dimension "d113" = 4.318
  dimension "d114" = 4.318
  dimension "d115" = 4.318
  constraint horizontal L0
  constraint vertical L1
  constraint vertical L2
  constraint horizontal L3
  constraint coincident L0.start L2
  constraint coincident L0 L3.end
  constraint coincident L3.end L1
  constraint coincident P2 L6
  constraint coincident P2 L8
  constraint tangent L6 A4
  constraint tangent L8 A4
  constraint coincident P4 L7
  constraint coincident P4 L8
  constraint tangent L7 A5
  constraint tangent L8 A5
  constraint equal A4 A5
  constraint coincident P3 L7
  constraint coincident P1 L6
  constraint coincident P2 L9.start
  constraint coincident P4 L9.end
  constraint collinear L14 L15
  constraint coincident P5 L10
  constraint coincident P5 L15
  constraint tangent L10 A12
  constraint tangent L15 A12
  constraint tangent L12 A13
  constraint tangent L15 A13
  constraint equal A12 A13
  constraint tangent L13 A14
  constraint tangent L14 A14
  constraint equal A12 A14
  constraint coincident P6 L11
  constraint coincident P6 L14
  constraint tangent L11 A15
  constraint tangent L14 A15
  constraint equal A12 A15
  constraint coincident A6.centre L16.start
  constraint parallel L8 L16
  constraint coincident A7.centre L17.start
  constraint coincident A10.centre L17.end
  constraint parallel L11 L17
  constraint vertical L18
  constraint coincident A1.centre A18.centre
  constraint coincident L8 L18.end
  constraint coincident L17 L19.end
  constraint perpendicular L17 L19
  constraint coincident L19.end A21.centre
  constraint parallel L16 L20
  measures "d11" diameter of A0
  measures "d14" diameter of A1
  measures "d15" distance of A0.centre A2.centre
  measures "d16" diameter of A2
  measures "d17" distance of A1.centre A3.centre
  measures "d18" diameter of A3
  measures "d49" distance of P1 P2
  measures "d51" distance of P3 P4
  measures "d52" radius of A4
  measures "d54" diameter of A6
  measures "d66" diameter of A7
  measures "d82" diameter of A8
  measures "d84" diameter of A9
  measures "d86" diameter of A10
  measures "d88" diameter of A11
  measures "d89" distance of L6.start P5
  measures "d90" distance of L7.start P6
  measures "d93" radius of A12
  measures "d110" distance of A6.centre L16.end
  measures "d112" diameter of A18
  measures "d113" diameter of A19
  measures "d114" diameter of A20
  measures "d115" diameter of A21
sketch "Sketch2" plane through (0, 0, 0) normal (0, 0, 1) x (1, 0, 0)
  line L0 (-41.8969, 27.5037) -> (4.7492, 27.5037)
  line L1 (4.7492, 27.5037) -> (4.7492, 14.7406)
  line L2 (-41.8969, 27.5037) -> (-41.8969, 14.7406)
  line L3 (-41.8969, 14.7406) -> (4.7492, 14.7406)
  constraint horizontal L0
  constraint perpendicular L0 L1
  constraint perpendicular L0 L2
  constraint perpendicular L1 L3
extrude "Extrude4" add sketch "Sketch1" along normal blind 4.7625 contours L0 L1 L2 L3 A1 L4 L5 L6 L8 A4 L9 L10 L12 L15 A12 A13 A18 A19 A20 L18 L20 | L1 A1 L7 L8 A5 L9 L11 L13 L14 A14 A15 A18 A19 A20 L18 L20 | A16 L16 | A16 L16 | A17 makes body 1
sketch "Sketch3" plane through (0, 0, 4.7625) normal (0, 0, 1) x (-1, 0, 0)
  circle A0 centre (-6.0728, -19.9051) radius 2.159
  circle A1 centre (-18.7728, -19.9051) radius 2.159
  circle A2 centre (-4.9703, -32.6051) radius 2.159
  circle A3 centre (57.4272, -19.9053) radius 2.159
  circle A4 centre (44.7272, -19.9053) radius 2.159
  circle A5 centre (43.6297, -42.4053) radius 2.159
  circle A6 centre (57.4272, -67.8053) radius 2.159
  circle A7 centre (-18.7728, -67.8053) radius 2.159
  circle A8 centre (43.6297, -32.6053) radius 2.159
  circle A9 centre (-4.9703, -42.4051) radius 2.159
  line L0 (39.3297, -47.5051) -> (-0.6703, -47.5051)
  line L1 (-0.6703, -47.5051) -> (-0.6703, -17.3451)
  arc A10 (-0.6703, -17.3451) -> (-3.2103, -14.8051) centre (-3.2103, -17.3451) ccw
  line L2 (-3.2103, -14.8051) -> (-19.7203, -14.8051)
  arc A11 (-19.7203, -14.8051) -> (-22.2603, -17.3451) centre (-19.7203, -17.3451) ccw
  line L3 (-22.2603, -17.3451) -> (-22.2603, -69.4151)
  arc A12 (-22.2603, -69.4151) -> (-19.7203, -71.9551) centre (-19.7203, -69.4151) ccw
  line L4 (-19.7203, -71.9551) -> (58.3797, -71.9551)
  arc A13 (58.3797, -71.9551) -> (60.9197, -69.4151) centre (58.3797, -69.4151) ccw
  line L5 (60.9197, -69.4151) -> (60.9197, -17.3451)
  arc A14 (60.9197, -17.3451) -> (58.3797, -14.8051) centre (58.3797, -17.3451) ccw
  line L6 (58.3797, -14.8051) -> (41.8697, -14.8051)
  arc A15 (41.8697, -14.8051) -> (39.3297, -17.3451) centre (41.8697, -17.3451) ccw
  line L7 (39.3297, -17.3451) -> (39.3297, -47.5051)
  line L8 (-0.6703, -27.5033) -> (-19.7213, -27.5033)
  line L9 (-0.6703, -27.5033) -> (58.3797, -27.5033)
  line L10 (60.9197, -24.9633) -> (60.9197, -17.3433)
  line L11 (58.3797, -14.8033) -> (-19.7243, -14.8033)
  line L12 (-22.2643, -17.3443) -> (-22.2613, -24.9643)
  arc A16 (58.3797, -27.5033) -> (60.9197, -24.9633) centre (58.3797, -24.9633) ccw
  arc A17 (-22.2613, -24.9643) -> (-19.7213, -27.5033) centre (-19.7213, -24.9633) ccw
  arc A18 (60.9197, -17.3433) -> (58.3797, -14.8033) centre (58.3797, -17.3433) ccw
  arc A19 (-19.7243, -14.8033) -> (-22.2643, -17.3443) centre (-19.7243, -17.3433) ccw
  circle A20 centre (-18.7728, -42.4051) radius 2.159
  point P0 (60.9197, -27.5033)
  point P1 (60.9197, -14.8033)
  point P2 (-22.2653, -14.8033)
  dimension "d96" = 12.7
  dimension "d97" = 83.185
  dimension "d98" = 2.54
  dimension "d99" = 2.54
  constraint coincident L1 L8.start
  constraint perpendicular L3 L8
  constraint coincident L5 P0
  constraint perpendicular L5 L9
  constraint perpendicular L9 L10
  constraint perpendicular L10 L11
  constraint coincident P0 L9
  constraint coincident P0 L10
  constraint tangent L9 A16
  constraint tangent L10 A16
  constraint tangent L8 A17
  constraint tangent L12 A17
  constraint equal A16 A17
  constraint coincident P1 L10
  constraint coincident P1 L11
  constraint tangent L10 A18
  constraint tangent L11 A18
  constraint coincident P2 L11
  constraint coincident P2 L12
  constraint tangent L11 A19
  constraint tangent L12 A19
  constraint equal A18 A19
  measures "d96" distance of P0 P1
  measures "d97" distance of P1 P2
  measures "d98" radius of A16
  measures "d99" radius of A18
extrude "Extrude5" add sketch "Sketch3" along normal blind 4.7625 separate body contours L1 A10 A15 L7 L9 L11 | L5 A14 L6 A15 L7 L9 L10 L11 A16 A18 | L1 A10 L2 A11 L3 L8 L11 A17 | A11 L3 L12 A19 makes body 2
fillet "Fillet5" radius 0.254 28 edges at (-19.3297, 47.5051, 4.7625) (0.6703, 32.4251, 4.7625) (1.4142, 15.549, 4.7625) (11.4653, 14.8051, 4.7625) (21.5163, 15.549, 4.7625) (22.2603, 43.3801, 4.7625) (21.5163, 71.2111, 4.7625) (-19.3297, 71.9551, 4.7625) (-60.1758, 71.2111, 4.7625) (-60.9197, 43.3801, 4.7625) (-60.1758, 15.549, 4.7625) (-50.1247, 14.8051, 4.7625) (-40.0737, 15.549, 4.7625) (-39.3297, 32.4251, 4.7625) (-19.3297, 47.5051, 0) (0.6703, 32.4251, 0) (1.4142, 15.549, 0) (11.4653, 14.8051, 0) (21.5163, 15.549, 0) (22.2603, 43.3801, 0) (21.5163, 71.2111, 0) (-19.3297, 71.9551, 0) (-60.1758, 71.2111, 0) (-60.9197, 43.3801, 0) (-60.1758, 15.549, 0) (-50.1247, 14.8051, 0) (-40.0737, 15.549, 0) (-39.3297, 32.4251, 0) on bodies 1
fillet "Fillet6" radius 0.254 24 edges at (-50.1247, 14.8051, 4.7625) (-50.1247, 14.8051, 9.525) (-60.1758, 15.549, 4.7625) (-60.1758, 15.549, 9.525) (-19.3297, 14.8042, 4.7625) (-19.3297, 14.8042, 9.525) (-60.9197, 21.1542, 4.7625) (-60.1758, 26.7594, 4.7625) (-48.8547, 27.5033, 4.7625) (-60.9197, 21.1542, 9.525) (-60.1758, 26.7594, 9.525) (-48.8547, 27.5033, 9.525) (11.4653, 14.8051, 4.7625) (11.4653, 14.8051, 9.525) (-19.3297, 27.5033, 4.7625) (-19.3297, 27.5033, 9.525) (21.5177, 15.5504, 4.7625) (21.5177, 15.5504, 9.525) (10.1958, 27.5033, 4.7625) (21.517, 26.7597, 4.7625) (22.2603, 21.1547, 4.7625) (10.1958, 27.5033, 9.525) (21.517, 26.7597, 9.525) (22.2603, 21.1547, 9.525) on bodies 2
equation "d94 = ( 3 / 16 ) * 1 in"
equation "d100 = ( 3 / 16 ) * 1 in"
named bodies: "ServoMount", "ServoBar"

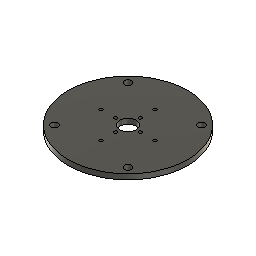
design "Winch1"
Autodesk Fusion 360 part; units mm, degrees
sketch "Sketch1" plane through (0, 0, 0) normal (0, 0, 1) x (1, 0, 0)
  circle A0 centre (0, 0) radius 7.5
  circle A1 centre (16.5, 0) radius 0.9375
  circle A2 centre (-16.5, 0) radius 0.9375
  circle A3 centre (0, -16.5) radius 0.9375
  circle A4 centre (0, 16.5) radius 0.9375
  line L0 (0, 0) -> (18.2563, 0) construction
  circle A5 centre (22.4506, 22.4506) radius 2.159
  circle A6 centre (22.4506, -22.4506) radius 2.159
  circle A7 centre (-22.4506, -22.4506) radius 2.159
  circle A8 centre (-22.4506, 22.4506) radius 2.159
  circle A9 centre (0, 0) radius 5
  circle A10 centre (0, 0) radius 36.5125
  line L1 (0, 0) -> (22.4506, 22.4506)
  line L2 (0, 0) -> (21.082, 0) construction
  line L3 (0, 0) -> (22.4506, -22.4506)
  line L4 (0, 0) -> (21.082, 0) construction
  line L5 (0, 0) -> (-22.4506, -22.4506)
  line L6 (0, 0) -> (21.082, 0) construction
  line L7 (0, 0) -> (-22.4506, 22.4506)
  line L8 (0, 0) -> (21.082, 0) construction
  arc A11 (-20.873, 23.9245) -> (20.873, 23.9245) centre (0, 0) ccw
  line L9 (16.5, 0) -> (10.5, 0)
  circle A12 centre (0, 0) radius 5.2451
  circle A13 centre (7.5, 0) radius 0.9375
  circle A14 centre (0, 7.5) radius 0.9375
  circle A15 centre (-7.5, 0) radius 0.9375
  circle A16 centre (0, -7.5) radius 0.9375
  dimension "d2" = 15
  dimension "d6" = 1.875
  dimension "d7" = 1.875
  dimension "d8" = 1.875
  dimension "d9" = 1.875
  dimension "d16" = 4.318
  dimension "d17" = 4.318
  dimension "d18" = 4.318
  dimension "d19" = 4.318
  dimension "d21" = 10
  dimension "d24" = 73.025
  dimension "d25" = 63.5
  dimension "d26" = 45
  dimension "d27" = 45
  dimension "d28" = 135
  dimension "d29" = 135
  dimension "d31" = 6
  dimension "d32" = 10.4902
  dimension "d33" = 1.875
  dimension "d35" = 360
  constraint coincident A0.centre L0.start
  constraint horizontal L0
  constraint concentric A10 A11
  constraint horizontal L2
  constraint coincident A5.centre A11
  constraint coincident A5.centre L1.end
  constraint horizontal L4
  constraint coincident A6.centre A11
  constraint coincident A6.centre L3.end
  constraint horizontal L6
  constraint coincident A7.centre A11
  constraint coincident A7.centre L5.end
  constraint horizontal L8
  constraint coincident A8.centre A11
  constraint coincident A8.centre L7.end
  constraint coincident A5 A11.end
  constraint coincident A8 A11.start
  constraint coincident A1.centre L9.start
  constraint coincident L0 L9.end
  constraint coincident L6 L9.end
  constraint concentric A0 A12
  constraint coincident L2 A13.centre
  constraint coincident A0 A13.centre
  measures "d2" diameter of A0
  measures "d6" diameter of A1
  measures "d7" diameter of A2
  measures "d8" diameter of A3
  measures "d9" diameter of A4
  measures "d16" diameter of A5
  measures "d17" diameter of A6
  measures "d18" diameter of A7
  measures "d19" diameter of A8
  measures "d21" diameter of A9
  measures "d24" diameter of A10
  measures "d25" diameter of A11
  measures "d26" angle of L1 L2
  measures "d27" angle of L3 L4
  measures "d28" angle of L5 L6
  measures "d29" angle of L7 L8
  measures "d31" distance of A1.centre L9.end
  measures "d32" diameter of A12
  measures "d33" diameter of A13
extrude "Extrude1" add sketch "Sketch1" along normal blind 3.175 contours A0 L1 L3 A12 A13 | A0 A5 A6 L1 L3 A11 A13 | A0 L1 L7 A12 A14 | A0 A6 A7 L3 L5 A11 A16 | A0 L3 L5 A12 A16 | A9 L1 L3 A12 | A9 L1 L7 A12 | A9 L3 L5 A12 | A0 L5 L7 A12 A15 | A9 L5 L7 A12 | A0 A7 A8 L5 L7 A11 A15 | A10
equation "d22 = ( 1 / 8 ) * 1 in"
named bodies: "Winch1"

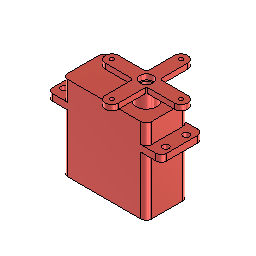
design "TD-8135MG Servo"
Autodesk Fusion 360 part; units mm, degrees